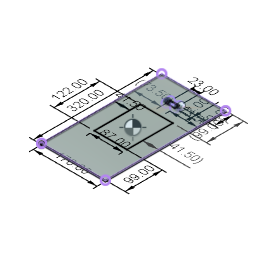
Bodemplaat v1 (Autodesk Fusion 360 design; units mm, degrees)
Autodesk Fusion 360 part; units mm, degrees
sketch "Sketch1" plane through (0, 0, 0) normal (0, 0, 1) x (1, 0, 0)
  line L0 (0, 0) -> (170, 0)
  line L1 (170, 0) -> (170, 320)
  line L2 (170, 320) -> (0, 320)
  line L3 (0, 320) -> (0, 0)
  dimension "d1" = 170
  dimension "d2" = 320
  constraint horizontal L0
  constraint vertical L1
  constraint horizontal L2
  constraint vertical L3
  constraint coincident L0.start L3.end
  measures "d1" distance of L0.start L0.end
  measures "d2" distance of L0.start L2.end
extrude "Extrude1" add sketch "Sketch1" along normal blind 3
sketch "Sketch2" plane through (0, 0, 3) normal (0, 0, 1) x (-1, 0, 0)
  line L0 (0, -320) -> (0, 0)
  line L1 (0, 0) -> (-170, 0)
  line L2 (-170, 0) -> (-170, -320)
  line L3 (-170, -320) -> (0, -320)
  line L4 (-73.5, -270) -> (-96.5, -270)
  line L5 (-96.5, -270) -> (-96.5, -258)
  line L6 (-96.5, -258) -> (-73.5, -258)
  line L7 (-73.5, -258) -> (-73.5, -270)
  dimension "d8" = 23
  dimension "d9" = 12
  dimension "d10" = 73.5
  dimension "d12" = 73.5
  dimension "d13" = 50
  constraint horizontal L4
  constraint vertical L5
  constraint horizontal L6
  constraint vertical L7
  measures "d8" distance of L4.start L4.end
  measures "d9" distance of L4.end L5.end
  measures "d10" distance of L2 L5
  measures "d12" distance of L0 L7
  measures "d13" distance of L3 L4
extrude "Extrude2" cut sketch "Sketch2" against normal blind 3 contours L4 L5 L6 L7
sketch "dd" plane through (0, 0, 3) normal (0, 0, 1) x (-1, 0, 0)
  line L0 (-41.5, -99) -> (-128.5, -99)
  line L1 (-128.5, -99) -> (-128.5, -221)
  line L2 (-128.5, -221) -> (-41.5, -221)
  line L3 (-41.5, -221) -> (-41.5, -99)
  line L4 (0, -320) -> (0, 0)
  line L5 (-170, 0) -> (-170, -320)
  line L6 (0, 0) -> (-170, 0)
  line L7 (-170, -320) -> (0, -320)
  dimension "d16" = 122
  dimension "d17" = 87
  dimension "d18" = 41.5
  dimension "d19" = 41.5
  dimension "d20" = 99
  dimension "d21" = 99
  constraint horizontal L0
  constraint vertical L1
  constraint horizontal L2
  constraint vertical L3
  measures "d16" distance of L0.start L2.end
  measures "d17" distance of L0.start L0.end
  measures "d18" distance of L3 L4
  measures "d19" distance of L1 L5
  measures "d20" distance of L0 L6
  measures "d21" distance of L2 L7
sketch "Sketch6" plane through (0, 0, 3) normal (0, 0, 1) x (-1, 0, 0)
  circle A0 centre (-99, -264) radius 1.5
  line L0 (-96.5, -270) -> (-96.5, -258)
  circle A1 centre (-99, -274) radius 1.5
  circle A2 centre (-71, -264) radius 1.5
  line L1 (-73.5, -258) -> (-73.5, -270)
  dimension "d22" = 2.5
  dimension "d23" = 3
  dimension "d24" = 6
  dimension "d26" = 3
  dimension "d27" = 2.5
  dimension "d28" = 6
  measures "d22" distance of A0.centre L0
  measures "d23" diameter of A0
  measures "d24" vertical distance of A0.centre L0.start
  measures "d26" diameter of A2
  measures "d27" distance of A2.centre L1
  measures "d28" vertical distance of A2.centre L1.end
hole "Hole1" at (71, 264, 3) direction (0, 0, -1) diameter 3 depth 3 tip angle 118
hole "Hole2" at (99, 274, 3) direction (0, 0, -1) diameter 3 depth 3 tip angle 118
